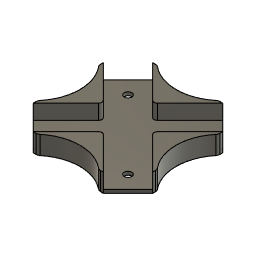
X500 Centerplate v1 (Autodesk Fusion 360 design; units mm, degrees)
Autodesk Fusion 360 part; units mm, degrees
sketch "Skizze1" plane through (0, 0, 0) normal (0, 1, 0) x (1, 0, 0)
  line L0 (-26.0309, 15.2828) -> (-26.0309, -15.2828)
  line L1 (-26.0309, -15.2828) -> (-15.2828, -26.0309)
  line L2 (-15.2828, -26.0309) -> (15.2828, -26.0309)
  line L3 (15.2828, -26.0309) -> (26.0309, -15.2828)
  line L4 (26.0309, -15.2828) -> (26.0309, 15.2828)
  line L5 (26.0309, 15.2828) -> (15.2828, 26.0309)
  line L6 (15.2828, 26.0309) -> (-15.2828, 26.0309)
  line L7 (-15.2828, 26.0309) -> (-26.0309, 15.2828)
  circle A0 centre (-15, 15) radius 1.65
  line L8 (0, 26.0309) -> (0, -26.0309) construction
  line L9 (-26.0309, 0) -> (26.0309, 0) construction
  circle A1 centre (15, 15) radius 1.65
  circle A2 centre (15, -15) radius 1.65
  circle A3 centre (-15, -15) radius 1.65
  line L10 (-26.0309, 15.2828) -> (-10.748, 0)
  line L11 (-10.748, 0) -> (-26.0309, -15.2828)
  line L12 (-15.2828, 26.0309) -> (0, 10.748)
  line L13 (0, 10.748) -> (15.2828, 26.0309)
  line L14 (26.0309, 15.2828) -> (10.748, 0)
  line L15 (10.748, 0) -> (26.0309, -15.2828)
  line L16 (15.2828, -26.0309) -> (0, -10.748)
  line L17 (-15.2828, -26.0309) -> (0, -10.748)
  arc A4 (-26.0309, -13.2828) -> (-26.0309, 13.2828) centre (-40.983, 0) ccw
  arc A5 (13.2828, -26.0309) -> (-13.2828, -26.0309) centre (0, -40.983) ccw
  arc A6 (26.0309, 13.2828) -> (26.0309, -13.2828) centre (40.983, 0) ccw
  arc A7 (-13.2828, 26.0309) -> (13.2828, 26.0309) centre (0, 40.983) ccw
  dimension "d1" = 15.2
  dimension "d2" = 3.3
  dimension "d3" = 8
  dimension "d4" = 15
  dimension "d5" = 15
  dimension "d6" = 45
  dimension "d7" = 2
  dimension "d8" = 2
  dimension "d10" = 20
  dimension "d12" = 360
  constraint horizontal L6
  constraint equal L5 L7
  constraint equal L1 L7
  constraint equal L3 L7
  constraint midpoint L6 L8.start
  constraint midpoint L2 L8.end
  constraint perpendicular L2 L8
  constraint parallel L3 L7
  constraint parallel L1 L5
  constraint parallel L0 L4
  constraint vertical L4
  constraint horizontal L2
  constraint equal L4 L6
  constraint midpoint L0 L9.start
  constraint midpoint L4 L9.end
  constraint coincident origin L8
  constraint coincident origin L9
  constraint symmetric A0 L8 A1
  constraint symmetric A0 L9 A3
  constraint symmetric L9 A1 A2
  constraint coincident L9 L10.end
  constraint perpendicular L7 L10
  constraint coincident L8 L12.end
  constraint perpendicular L7 L12
  constraint coincident L9 L14.end
  constraint perpendicular L5 L14
  constraint coincident L8 L16.end
  constraint perpendicular L3 L16
  constraint coincident L0 A4.start
  constraint coincident L0 A4.end
  measures "d1" distance of L0.start L6.end
  measures "d2" diameter of A0
  measures "d3" distance of L7 A0.centre
  measures "d4" horizontal distance of origin A0.centre
  measures "d5" vertical distance of origin A0.centre
  measures "d6" angle of L6 L7
  measures "d7" distance of L0.start A4.end
  measures "d8" distance of L0.end A4.start
  measures "d10" radius of A4
extrude "Extrusion1" add sketch "Skizze1" along normal blind 1.5 contours L0 L10 L11 A4 | L1 L3 L5 L7 L10 L11 L12 L13 L14 L15 L16 L17 | L6 L12 L13 A7 | L2 L16 L17 A5 | L4 L14 L15 A6
extrude "Extrusion2" add sketch "Skizze1" along normal blind 8 contours L0 L10 L11 A4 | L6 L12 L13 A7 | L2 L16 L17 A5 | L4 L14 L15 A6
fillet "Abrundung1" radius 1.5 4 edges at (0, 4.75, -10.748) (10.748, 4.75, 0) (0, 4.75, 10.748) (-10.748, 4.75, 0)
fillet "Abrundung3" radius 2 8 edges at (-26.0309, 4, 13.2828) (-26.0309, 4, -13.2828) (-13.2828, 4, 26.0309) (13.2828, 4, 26.0309) (26.0309, 4, 13.2828) (26.0309, 4, -13.2828) (13.2828, 4, -26.0309) (-13.2828, 4, -26.0309)
equation "d8 = d7"
